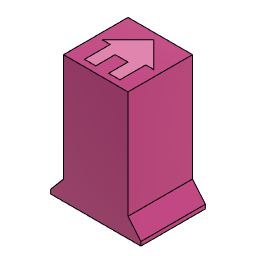
Key_Home (Autodesk Fusion 360 design; units mm, degrees)
Autodesk Fusion 360 part; units mm, degrees
sketch "Skizze1" plane through (0, 0, 0) normal (0, 0, 1) x (1, 0, 0)
sketch "Skizze1 (2)" plane through (0, 0, 0) normal (0, 0, 1) x (1, 0, 0) in component "Key_Home"
  line L0 (5, -5) -> (-5, -5)
  line L1 (-5, -5) -> (-5, 5)
  line L2 (-5, 5) -> (5, 5)
  line L3 (5, 5) -> (5, -5)
  line L4 (5, -5) -> (-5, 5) construction
  line L5 (-5, -5) -> (5, 5) construction
  dimension "d1" = 10
  dimension "d2" = 10
  constraint horizontal L0
  constraint perpendicular L0 L1
  constraint parallel L0 L2
  constraint parallel L1 L3
  constraint coincident L4 origin
  constraint coincident L5 origin
  measures "d1" distance of L1.end L2.end
  measures "d2" distance of L0.end L1.end
extrude "Extrusion1" add sketch "Skizze1 (2)" along normal blind 19.7 makes body 1 in component "Key_Home"
sketch "Skizze2" plane through (0, 0, 19.7) normal (0, 0, 1) x (-1, 0, 0) in component "Key_Home"
  line L0 (-5, -5) -> (5, -5)
  line L1 (5, -5) -> (5, 5)
  line L2 (5, 5) -> (-5, 5)
  line L3 (-5, 5) -> (-5, -5)
  line L4 (2.75, 4) -> (1, 4)
  line L5 (1, 4) -> (1, 1)
  line L6 (1, 1) -> (-1, 1)
  line L7 (-1, 1) -> (-1, 4)
  line L8 (-1, 4) -> (-2.75, 4)
  line L9 (-2.75, 4) -> (-2.75, 0)
  line L10 (-2.75, 0) -> (-4, 0)
  line L11 (-4, 0) -> (0, -4)
  line L12 (0, -4) -> (4, 0)
  line L13 (4, 0) -> (2.75, 0)
  line L14 (2.75, 0) -> (2.75, 4)
  dimension "d5" = 1
  dimension "d6" = 1
  dimension "d7" = 1
  dimension "d8" = 1.25
  dimension "d11" = 2
  dimension "d12" = 3
  dimension "d13" = 5
  constraint horizontal L4
  constraint perpendicular L4 L5
  constraint perpendicular L5 L6
  constraint perpendicular L6 L7
  constraint parallel L7 L9
  constraint perpendicular L7 L10
  constraint perpendicular L7 L13
  constraint perpendicular L4 L14
  constraint perpendicular L7 L8
  constraint equal L4 L8
  constraint equal L10 L13
  constraint equal L11 L12
  constraint equal L9 L14
  constraint equal L5 L7
  constraint vertical origin L11.end
  measures "d5" distance of L0 L11.end
  measures "d6" distance of L1 L12.end
  measures "d7" distance of L2 L4
  measures "d8" distance of L12.end L13.end
  measures "d11" distance of L5 L7
  measures "d12" distance of L4.end L5.end
  measures "d13" distance of L0 L13
extrude "Extrusion2" cut sketch "Skizze2" against normal blind 0.5 contours L4 L5 L6 L7 L8 L9 L10 L11 L12 L13 L14 bodies 1 in component "Key_Home"
extrude "Extrusion1'" add 1 faces at (0, 0.6667, 19.2) along direction (0, 0, 1) up to surface (0.5 mm away) separate body on bodies 1 makes body 2 in component "Key_Home_Icon"
sketch "Skizze3" plane through (0, -5, 0) normal (0, -1, 0) x (1, 0, 0) in component "Key_Home"
  line L0 (-5, 0) -> (5, 0)
  line L1 (5, 0) -> (5, 19.7)
  line L2 (5, 19.7) -> (-5, 19.7)
  line L3 (-5, 19.7) -> (-5, 0)
  line L4 (5, 0) -> (7, 0)
  line L5 (7, 0) -> (7, 0.6165)
  line L6 (7, 0.6165) -> (5, 3)
  line L7 (0, 20) -> (0, 2.5)
  line L8 (-7, 0) -> (-7, 0.6165)
  line L9 (-7, 0.6165) -> (-5, 3)
  line L10 (-5, 0) -> (-7, 0)
  point P0 (-5, 0)
  dimension "d18" = 2
  dimension "d19" = 3
  dimension "d20" = 40
  constraint coincident L0.end L1.start
  constraint perpendicular L1 L4
  constraint perpendicular L4 L5
  constraint coincident L1 L6.end
  constraint symmetric L0.end L7 P0
  constraint symmetric L4.end L7 L8.start
  constraint symmetric L5.end L7 L8.end
  constraint symmetric L6.end L7 L9.end
  measures "d18" distance of L0.end L4.end
  measures "d19" distance of L0.end L6.end
  measures "d20" angle of L1 L6
extrude "Extrusion3" add sketch "Skizze3" against normal up to surface (10 mm away) contours L3 L8 L9 L10 | L1 L4 L5 L6 bodies 1 in component "Key_Home"
component "Key_Home" placed x (1, 0, 0) y (0, 1, 0) z (0, 0, 1) at (0, 0, 0)
component "Key_Home_Icon" placed x (1, 0, 0) y (0, 1, 0) z (0, 0, 1) at (0, 0, 0)
equation "d3 = 21.7 mm - 2 mm"
equation "d6 = d5"
equation "d7 = d5"
equation "d19 = 5 mm - 2 mm"
